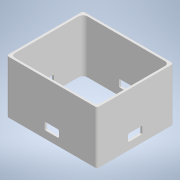
# Autodesk Inventor part: beer crate
Saved by Autodesk Inventor 2022.2 (Build 262287010, 287A)
## iProperties
Created: 2022-03-18
Part Number: beer crate
Material: Generic
Document SubType Name: Modeling
Designer: Finn Oriwohl
Mass: 3673.69 g
Surface Area: 7478.73 cm^2
Volume: 3673.69 cm^3
Density: 1 g/cm^3
Appearance: Smooth - Dark Forest Green
Author: Finn Oriwohl
Autodesk Inventor part; units mm, degrees
ref_plane "YZ Plane" through (0, 0, 0) normal (1, 0, 0) x (0, 1, 0)
ref_plane "XZ Plane" through (0, 0, 0) normal (0, 1, 0) x (-1, 0, 0)
ref_plane "XY Plane" through (0, 0, 0) normal (0, 0, 1) x (1, 0, 0)
sketch "Sketch1" plane through (0, 0, 0) normal (0, 1, 0) x (-1, 0, 0)
  line L0 (-180, 167.5) -> (180, 167.5)
  line L1 (200, 147.5) -> (200, -147.5)
  line L2 (180, -167.5) -> (-180, -167.5)
  line L3 (-200, -147.5) -> (-200, 147.5)
  line L4 (-200, 167.5) -> (200, -167.5) construction
  line L5 (200, 167.5) -> (-200, -167.5) construction
  line L6 (-200, -177.5) -> (200, -177.5)
  line L7 (210, -167.5) -> (210, 167.5)
  line L8 (200, 177.5) -> (-200, 177.5)
  line L9 (-210, 167.5) -> (-210, -167.5)
  arc A0 (180, -167.5) -> (200, -147.5) centre (180, -147.5) ccw
  arc A1 (-200, -147.5) -> (-180, -167.5) centre (-180, -147.5) ccw
  arc A2 (-180, 167.5) -> (-200, 147.5) centre (-180, 147.5) ccw
  arc A3 (200, 147.5) -> (180, 167.5) centre (180, 147.5) ccw
  arc A4 (210, 167.5) -> (200, 177.5) centre (200, 167.5) ccw
  arc A5 (200, -177.5) -> (210, -167.5) centre (200, -167.5) ccw
  arc A6 (-210, -167.5) -> (-200, -177.5) centre (-200, -167.5) ccw
  arc A7 (-200, 177.5) -> (-210, 167.5) centre (-200, 167.5) ccw
  point P0 (0, 0)
  dimension "d0" = 400
  dimension "d1" = 335
  dimension "d2" = 10
  dimension "d3" = 20
  dimension "d4" = 20
  dimension "d5" = 10
  constraints: 20 end point, 16 point on circle, 16 tangent, 8 centre point, 8 point on line, 5 equal radius, 4 parallel, 2 midpoint, 2 perpendicular, 1 horizontal, 3 other
  measures "d0" distance of L4.end L5.end
  measures "d1" distance of L5.start L4.end
  measures "d2" distance between parallel lines of L2 L6
  measures "d3" radius of A0
  measures "d4" radius of A1
  measures "d5" radius of A4
extrude "Extrusion1" add sketch "Sketch1" against normal blind 245
sketch "Sketch2" plane through (-200, 0, 177.5) normal (0, 0, 1) x (1, 0, 0)
  line L0 (400, -245) -> (0, -245) projected
  line L1 (228, -177) -> (172, -177)
  line L2 (167, -182) -> (167, -206)
  line L3 (172, -211) -> (228, -211)
  line L4 (233, -206) -> (233, -182)
  line L5 (233, -177) -> (167, -211) construction
  line L6 (167, -177) -> (233, -211) construction
  line L7 (380, -245) -> (20, -245) projected
  line L8 (200, -245) -> (200, -168) construction
  arc A0 (172, -177) -> (167, -182) centre (172, -182) ccw
  arc A1 (233, -182) -> (228, -177) centre (228, -182) ccw
  arc A2 (228, -211) -> (233, -206) centre (228, -206) ccw
  arc A3 (167, -206) -> (172, -211) centre (172, -206) ccw
  point P0 (200, 0)
  point P1 (200, -194)
  point P2 (200, -194)
  dimension "d8" = 34
  dimension "d9" = 51
  dimension "d10" = 5
  constraints: 14 end point, 9 point on line, 8 point on circle, 8 tangent, 5 midpoint, 4 centre point, 3 equal radius, 2 parallel, 1 horizontal, 1 perpendicular, 1 vertical
  measures "d8" distance of L5.end L6.start
  measures "d9" distance of point (200, -194) point (200, -245)
  measures "d10" radius of A0
extrude "Extrusion2" cut sketch "Sketch2" against normal through all
sketch "Sketch3" plane through (210, 0, 167.5) normal (1, 0, 0) x (0, 0, -1)
  line L0 (195.5, -177) -> (139.5, -177)
  line L1 (134.5, -182) -> (134.5, -206)
  line L2 (139.5, -211) -> (195.5, -211)
  line L3 (200.5, -206) -> (200.5, -182)
  line L4 (200.5, -177) -> (134.5, -211) construction
  line L5 (134.5, -177) -> (200.5, -211) construction
  arc A0 (139.5, -177) -> (134.5, -182) centre (139.5, -182) ccw
  arc A1 (200.5, -182) -> (195.5, -177) centre (195.5, -182) ccw
  arc A2 (195.5, -211) -> (200.5, -206) centre (195.5, -206) ccw
  arc A3 (134.5, -206) -> (139.5, -211) centre (139.5, -206) ccw
  line L6 (335, -245) -> (0, -245) projected
  line L7 (167.5, -245) -> (167.5, -152) construction
  point P0 (167.5, 0)
  point P1 (167.5, -194)
  point P2 (167.5, -194)
  point P3 (167.5, -194)
  dimension "d13" = 34
  dimension "d14" = 51
  dimension "d15" = 5
  constraints: 14 end point, 9 point on line, 8 point on circle, 8 tangent, 5 midpoint, 4 centre point, 3 equal radius, 2 parallel, 1 horizontal, 1 perpendicular, 1 vertical
  measures "d13" distance of L4.end L5.start
  measures "d14" distance of point (167.5, -194) L7.start
  measures "d15" radius of A0
extrude "Extrusion3" cut sketch "Sketch3" against normal through all
equation "\"d3\" = d4"
body "Solid1"
